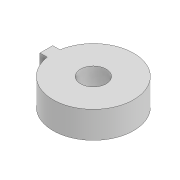
# Autodesk Inventor part: Test_gear_p2
Saved by Autodesk Inventor 2022 (Build 260153000, 153)
## iProperties
Created: 2022-07-12
Part Number: Test_gear_p2
Material: Generic
Document SubType Name: Modeling
Designer: dell
Density: 1 g/cm^3
Appearance: Default
Author: dell
Autodesk Inventor part; units mm, degrees
ref_plane "YZ Plane" through (0, 0, 0) normal (1, 0, 0) x (0, 1, 0)
ref_plane "XZ Plane" through (0, 0, 0) normal (0, 1, 0) x (-1, 0, 0)
ref_plane "XY Plane" through (0, 0, 0) normal (0, 0, 1) x (1, 0, 0)
sketch "Sketch1" plane through (0, 0, 0) normal (0, 1, 0) x (-1, 0, 0)
  circle A0 centre (0, 0) radius 4.7674
  circle A1 centre (0, 0) radius 15
  line L0 (14.8106, 2.3764) -> (14.8106, -2.3764)
  line L1 (14.8106, -2.3764) -> (17.5065, -2.3764)
  line L2 (17.5065, -2.3764) -> (17.5065, 2.3764)
  line L3 (17.5065, 2.3764) -> (14.8106, 2.3764)
  dimension "d0" = 30
  dimension "d1" = 9.5349
  constraints: 8 end point, 2 centre point, 2 coincident, 2 parallel, 2 point on circle, 1 perpendicular, 1 vertical
  measures "d0" diameter of A1
  measures "d1" diameter of A0
extrude "Extrusion1" add sketch "Sketch1" along normal blind 10
body "Solid1"
